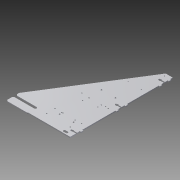
# Autodesk Inventor part: side_frame_v2
Saved by Autodesk Inventor 2013 (Build 170138000, 138)
## iProperties
Created: 2013-11-17
Part Number: side_frame_v2
Material: Generic
Document SubType Name: Modeling
Designer: Masta
Density: 1 g/cm^3
Author: Masta
Autodesk Inventor part; units mm, degrees
ref_plane "YZ Plane" through (0, 0, 0) normal (1, 0, 0) x (0, 1, 0)
ref_plane "XZ Plane" through (0, 0, 0) normal (0, 1, 0) x (-1, 0, 0)
ref_plane "XY Plane" through (0, 0, 0) normal (0, 0, 1) x (1, 0, 0)
sketch "Sketch1" plane through (0, 0, 0) normal (0, 0, 1) x (1, 0, 0)
  line L0 (255.7808, 350.0828) -> (255.7808, 358.8828)
  line L1 (251.6808, 67.29) -> (255.7808, 67.29)
  line L2 (255.7808, 67.29) -> (255.7808, 76.09)
  line L3 (255.7808, 76.09) -> (251.6808, 76.09)
  line L4 (251.6808, 76.09) -> (251.6808, 194.9901)
  line L5 (251.6808, 32.5401) -> (100.8808, 32.5401)
  line L6 (231.7439, 44.5401) -> (223.7479, 44.5401)
  line L7 (230.5808, 213.3401) -> (234.5808, 213.3401)
  line L8 (234.5808, 211.5401) -> (239.6808, 211.5401)
  line L9 (251.6808, 57.7345) -> (239.6808, 57.7345)
  line L10 (239.6808, 57.7345) -> (239.6808, 59.5345)
  line L11 (230.5808, 53.3345) -> (234.5808, 53.3345)
  line L12 (234.5808, 51.5345) -> (239.6808, 51.5345)
  line L13 (239.6808, 59.5345) -> (234.5808, 59.5345)
  line L14 (234.5808, 53.3345) -> (234.5808, 51.5345)
  line L15 (239.6808, 53.3345) -> (251.6808, 53.3345)
  line L16 (239.6808, 51.5345) -> (239.6808, 53.3345)
  line L17 (251.6808, 57.7345) -> (251.6808, 67.29)
  line L18 (251.6808, 217.7401) -> (239.6808, 217.7401)
  line L19 (255.7808, 236.0901) -> (251.6808, 236.0901)
  line L20 (251.6808, 236.0901) -> (251.6808, 350.0828)
  line L21 (255.7808, 203.7901) -> (251.6808, 203.7901)
  line L22 (251.6808, 194.9901) -> (255.7808, 194.9901)
  line L23 (255.7808, 194.9901) -> (255.7808, 203.7901)
  line L24 (251.6808, 227.2901) -> (251.6808, 217.7401)
  line L25 (251.6808, 213.3401) -> (251.6808, 203.7901)
  line L26 (251.6808, 382.3828) -> (255.7808, 382.3828)
  line L27 (255.7808, 382.3828) -> (255.7808, 391.1828)
  line L28 (255.7808, 391.1828) -> (251.6808, 391.1828)
  line L29 (251.6808, 391.1828) -> (251.6808, 400.5401)
  line L30 (255.7808, 358.8828) -> (251.6808, 358.8828)
  line L31 (251.6808, 350.0828) -> (255.7808, 350.0828)
  line L32 (73.8808, 35.5401) -> (73.8808, 51.1401)
  line L33 (239.6808, 211.5401) -> (239.6808, 213.3401)
  line L34 (230.5808, 217.7401) -> (230.5808, 213.3401)
  line L35 (73.8808, 77.5401) -> (226.2808, 400.5401)
  line L36 (234.5808, 217.7401) -> (230.5808, 217.7401)
  line L37 (234.5808, 217.7401) -> (234.5808, 219.5401)
  line L38 (251.6808, 400.5401) -> (226.2808, 400.5401)
  line L39 (239.6808, 213.3401) -> (251.6808, 213.3401)
  line L40 (231.7439, 36.5395) -> (223.7482, 36.5395)
  line L41 (239.6808, 219.5401) -> (234.5808, 219.5401)
  line L42 (98.8808, 30.5401) -> (78.8808, 30.5401)
  line L43 (234.5808, 213.3401) -> (234.5808, 211.5401)
  line L44 (230.5808, 372.825) -> (230.5808, 368.425)
  line L45 (234.5808, 372.825) -> (230.5808, 372.825)
  line L46 (234.5808, 372.825) -> (234.5808, 374.625)
  line L47 (251.6808, 372.825) -> (239.6808, 372.825)
  line L48 (230.5808, 368.425) -> (234.5808, 368.425)
  line L49 (239.6808, 368.425) -> (251.6808, 368.425)
  line L50 (234.5808, 366.625) -> (239.6808, 366.625)
  line L51 (239.6808, 374.625) -> (234.5808, 374.625)
  line L52 (234.5808, 368.425) -> (234.5808, 366.625)
  line L53 (251.6808, 372.825) -> (251.6808, 382.3828)
  line L54 (251.6808, 368.425) -> (251.6808, 358.8828)
  line L55 (230.5808, 57.7345) -> (230.5808, 53.3345)
  line L56 (234.5808, 57.7345) -> (230.5808, 57.7345)
  line L57 (234.5808, 57.7345) -> (234.5808, 59.5345)
  line L58 (239.6808, 366.625) -> (239.6808, 368.425)
  line L59 (239.6808, 372.825) -> (239.6808, 374.625)
  line L60 (78.8808, 56.1401) -> (148.8808, 56.1401)
  line L61 (78.8808, 56.1401) -> (73.8808, 51.1401)
  line L62 (78.8808, 64.9401) -> (148.8808, 64.9401)
  line L63 (73.8808, 69.9401) -> (73.8808, 77.5401)
  line L64 (78.8808, 64.9401) -> (73.8808, 69.9401)
  line L65 (251.6808, 227.2901) -> (255.7808, 227.2901)
  line L66 (255.7808, 227.2901) -> (255.7808, 236.0901)
  line L67 (239.6808, 217.7401) -> (239.6808, 219.5401)
  line L68 (78.8808, 30.5401) -> (73.8808, 35.5401)
  line L69 (100.8808, 32.5401) -> (98.8808, 30.5401)
  line L70 (251.6808, 32.5401) -> (251.6808, 53.3345)
  line L71 (136.6808, 189.5401) -> (231.6808, 189.5401) construction
  line L72 (231.6808, 189.5401) -> (231.6808, 93.5401) construction
  line L73 (231.6808, 93.5401) -> (136.6808, 93.5401) construction
  line L74 (136.6808, 93.5401) -> (136.6808, 189.5401) construction
  line L75 (164.6808, 93.5401) -> (208.6808, 93.5401) construction
  line L76 (208.6808, 93.5401) -> (208.6808, 187.5401) construction
  line L77 (208.6808, 187.5401) -> (164.6808, 187.5401) construction
  line L78 (164.6808, 187.5401) -> (164.6808, 93.5401) construction
  line L79 (160.3808, 93.5401) -> (208.6808, 93.5401) construction
  line L80 (208.6808, 93.5401) -> (208.6808, 168.5401) construction
  line L81 (208.6808, 168.5401) -> (160.3808, 168.5401) construction
  line L82 (160.3808, 168.5401) -> (160.3808, 93.5401) construction
  line L83 (208.6808, 168.5401) -> (208.6808, 174.8401) construction
  arc A0 (148.8808, 56.1401) -> (148.8808, 64.9401) centre (148.8808, 60.5401) ccw
  arc A1 (231.7439, 36.5395) -> (231.7439, 44.5401) centre (231.7439, 40.5398) ccw
  arc A2 (223.7479, 44.5401) -> (223.7482, 36.5395) centre (223.7482, 40.5398) ccw
  point P0 (0, 0)
  point P1 (219.7479, 40.5401)
  dimension "d0" = 177.8
  dimension "d9" = 95
  dimension "d10" = 96
  dimension "d11" = 44
  dimension "d12" = 94
  dimension "d15" = 48.3
  dimension "d16" = 75
  dimension "d18" = 6.3
  dimension "d19" = 23
  dimension "d20" = 20
  dimension "d21" = 63
  dimension "d22" = 4.1
  dimension "d23" = 8.8
  constraints: 168 end point, 17 collinear, 11 coincident, 7 parallel, 7 point on circle, 5 tangent, 4 horizontal, 3 centre point, 3 perpendicular, 1 vertical
  measures "d0" distance between parallel lines of L32 L70
  measures "d9" distance of L72.end L73.end
  measures "d10" distance of L71.end L72.end
  measures "d11" distance of L77.end L76.end
  measures "d12" distance of L75.end L76.end
  measures "d15" distance of L81.end L80.end
  measures "d16" distance of L80.end L75.end
  measures "d18" distance of L80.end L83.end
  measures "d19" distance between parallel lines of L72 L80
  measures "d20" distance between parallel lines of L4 L72
  measures "d21" distance between parallel lines of L42 L73
  measures "d22" distance between parallel lines of L2 L17
  measures "d23" distance of L1.end L2.end
extrude "Extrusion1" add sketch "Sketch1" against normal blind 4
hole "Hole1" at (136.6808, 189.5401, 0) at (136.6808, 93.5401, 0) at (231.6808, 93.5401, 0) at (231.6808, 189.5401, 0) at (160.3808, 93.5401, 0) at (208.6808, 93.5401, 0) at (208.6808, 174.8401, 0) at (160.3808, 168.5401, 0) at (164.6808, 93.5401, 0) at (164.6808, 187.5401, 0) at (208.6808, 187.5401, 0) direction (0, 0, -1) diameter 3.6 end through all
sketch "Sketch2" plane through (0, 0, 0) normal (0, 0, 1) x (1, 0, 0)
  line L0 (78.8808, 64.9401) -> (148.8808, 64.9401) projected
  line L1 (251.6808, 76.09) -> (251.6808, 194.9901) projected
  line L2 (162.1808, 84.5401) -> (212.1808, 84.5401) construction
  line L3 (212.1808, 84.5401) -> (212.1808, 234.5401) construction
  line L4 (212.1808, 234.5401) -> (162.1808, 234.5401) construction
  line L5 (162.1808, 234.5401) -> (162.1808, 84.5401) construction
  line L6 (162.1808, 84.5401) -> (212.1808, 234.5401) construction
  line L7 (212.1808, 84.5401) -> (162.1808, 234.5401) construction
  line L8 (129.6808, 49.5401) -> (244.6808, 49.5401) construction
  line L9 (244.6808, 49.5401) -> (244.6808, 269.5401) construction
  line L10 (244.6808, 269.5401) -> (129.6808, 269.5401) construction
  line L11 (129.6808, 269.5401) -> (129.6808, 49.5401) construction
  line L12 (129.6808, 49.5401) -> (244.6808, 269.5401) construction
  line L13 (244.6808, 49.5401) -> (129.6808, 269.5401) construction
  line L14 (223.7479, 44.5401) -> (231.7439, 44.5401) projected
  point P0 (0, 0)
  point P1 (187.1808, 159.5401)
  point P2 (187.1808, 159.5401)
  dimension "d33" = 50
  dimension "d34" = 150
  dimension "d35" = 115
  dimension "d36" = 220
  dimension "d38" = 7
  dimension "d82" = 5
  constraints: 24 end point, 5 midpoint, 4 coincident, 4 parallel, 2 horizontal, 2 perpendicular
  measures "d33" distance of L4.end L3.end
  measures "d34" distance of L3.end L2.end
  measures "d35" distance of L10.end L9.end
  measures "d36" distance of L9.end L8.end
  measures "d38" distance between parallel lines of L1 L9
  measures "d82" distance between parallel lines of L14 L8
hole "Hole2" at (162.1808, 234.5401, 0) at (162.1808, 84.5401, 0) at (212.1808, 84.5401, 0) at (212.1808, 234.5401, 0) direction (0, 0, -1) diameter 4.6 end through all
sketch "Sketch3" plane through (0, 0, 0) normal (0, 0, 1) x (1, 0, 0)
  line L0 (226.2808, 400.5401) -> (73.8808, 77.5401) projected
  line L1 (73.8808, 77.5401) -> (73.8808, 69.9401) projected
  line L2 (73.8808, 69.9401) -> (78.8808, 64.9401) projected
  line L3 (78.8808, 56.1401) -> (73.8808, 51.1401) projected
  line L4 (73.8808, 51.1401) -> (73.8808, 35.5401) projected
  line L5 (73.8808, 35.5401) -> (78.8808, 30.5401) projected
  line L6 (98.8808, 30.5401) -> (100.8808, 32.5401) projected
  line L7 (78.8808, 64.9401) -> (28.8808, 64.9401)
  line L8 (28.8808, 64.9401) -> (23.8808, 69.9401)
  line L9 (23.8808, 77.5401) -> (23.8808, 69.9401)
  line L10 (23.8808, 77.5401) -> (226.2808, 400.5401)
  line L11 (78.8808, 56.1401) -> (28.8808, 56.1401)
  line L12 (28.8808, 56.1401) -> (23.8808, 51.1401)
  line L13 (23.8808, 51.1401) -> (23.8808, 35.5401)
  line L14 (78.8808, 30.5401) -> (28.8808, 30.5401)
  line L15 (23.8808, 35.5401) -> (28.8808, 30.5401)
  point P0 (0, 0)
  point P1 (251.6808, 67.29)
  point P2 (251.6808, 76.09)
  point P3 (251.6808, 194.9901)
  point P4 (251.6808, 203.7901)
  point P5 (251.6808, 227.2901)
  point P6 (251.6808, 236.0901)
  point P7 (251.6808, 350.0828)
  point P8 (251.6808, 358.8828)
  point P9 (251.6808, 382.3828)
  point P10 (251.6808, 391.1828)
  dimension "d46" = 50
  dimension "d47" = 5
  dimension "d48" = 7.6
  constraints: 18 end point, 7 perpendicular
  measures "d46" distance of L2.end L7.end
  measures "d47" horizontal distance of L7.end L8.end
  measures "d48" distance of L9.start L8.end
extrude "Extrusion2" add sketch "Sketch3" against normal up to surface (4 mm away)
hole "Hole3" at (251.6808, 67.29, 0) at (251.6808, 76.09, 0) at (251.6808, 194.9901, 0) at (251.6808, 203.7901, 0) at (251.6808, 227.2901, 0) at (251.6808, 236.0901, 0) at (251.6808, 350.0828, 0) at (251.6808, 358.8828, 0) at (251.6808, 382.3828, 0) at (251.6808, 391.1828, 0) direction (0, 0, -1) diameter 1 end through all
sketch "Sketch5" plane through (0, 0, 0) normal (0, 0, 1) x (1, 0, 0)
  line L0 (251.6808, 53.3345) -> (239.6808, 53.3345) projected
  line L1 (239.6808, 53.3345) -> (239.6808, 51.5345) projected
  line L2 (239.6808, 51.5345) -> (234.5808, 51.5345) projected
  line L3 (234.5808, 51.5345) -> (234.5808, 53.3345) projected
  line L4 (234.5808, 53.3345) -> (230.5808, 53.3345) projected
  line L5 (230.5808, 53.3345) -> (230.5808, 57.7345) projected
  line L6 (230.5808, 57.7345) -> (234.5808, 57.7345) projected
  line L7 (234.5808, 57.7345) -> (234.5808, 59.5345) projected
  line L8 (234.5808, 59.5345) -> (239.6808, 59.5345) projected
  line L9 (239.6808, 59.5345) -> (239.6808, 57.7345) projected
  line L10 (239.6808, 57.7345) -> (251.6808, 57.7345) projected
  line L11 (251.6808, 213.3401) -> (239.6808, 213.3401) projected
  line L12 (239.6808, 213.3401) -> (239.6808, 211.5401) projected
  line L13 (239.6808, 211.5401) -> (234.5808, 211.5401) projected
  line L14 (234.5808, 211.5401) -> (234.5808, 213.3401) projected
  line L15 (234.5808, 213.3401) -> (230.5808, 213.3401) projected
  line L16 (230.5808, 213.3401) -> (230.5808, 217.7401) projected
  line L17 (230.5808, 217.7401) -> (234.5808, 217.7401) projected
  line L18 (234.5808, 217.7401) -> (234.5808, 219.5401) projected
  line L19 (234.5808, 219.5401) -> (239.6808, 219.5401) projected
  line L20 (239.6808, 219.5401) -> (239.6808, 217.7401) projected
  line L21 (239.6808, 217.7401) -> (251.6808, 217.7401) projected
  line L22 (251.6808, 368.425) -> (239.6808, 368.425) projected
  line L23 (239.6808, 368.425) -> (239.6808, 366.625) projected
  line L24 (239.6808, 366.625) -> (234.5808, 366.625) projected
  line L25 (234.5808, 366.625) -> (234.5808, 368.425) projected
  line L26 (234.5808, 368.425) -> (230.5808, 368.425) projected
  line L27 (230.5808, 368.425) -> (230.5808, 372.825) projected
  line L28 (230.5808, 372.825) -> (234.5808, 372.825) projected
  line L29 (234.5808, 372.825) -> (234.5808, 374.625) projected
  line L30 (234.5808, 374.625) -> (239.6808, 374.625) projected
  line L31 (239.6808, 374.625) -> (239.6808, 372.825) projected
  line L32 (239.6808, 372.825) -> (251.6808, 372.825) projected
  line L33 (231.7439, 36.5395) -> (223.7482, 36.5395) projected
  line L34 (251.6808, 217.7401) -> (251.6808, 213.3401)
  line L35 (251.6808, 368.425) -> (251.6808, 372.825)
  line L36 (251.6808, 53.3345) -> (251.6808, 57.7345)
  line L37 (28.8808, 64.9401) -> (148.8808, 64.9401) projected
  arc A0 (148.8808, 56.1401) -> (148.8808, 64.9401) centre (148.8808, 60.5401) ccw projected
  line L38 (148.8808, 56.1401) -> (28.8808, 56.1401) projected
  arc A1 (98.8808, 56.1401) -> (98.8808, 64.9401) centre (98.8808, 60.5401) ccw
  point P0 (0, 0)
  point P1 (251.6808, 215.5401)
  point P2 (251.6808, 370.625)
  point P3 (251.6808, 55.5345)
  dimension "d85" = 50
  constraints: 6 end point, 3 midpoint, 2 collinear, 2 point on circle, 2 point on line, 2 tangent, 1 centre point, 1 perpendicular
  measures "d85" distance of A0.centre A1.centre
extrude "Extrusion3" add sketch "Sketch5" against normal up to surface (4 mm away)
sketch "Sketch6" plane through (0, 0, 0) normal (0, 0, 1) x (1, 0, 0)
  line L0 (251.6808, 204.2901) -> (251.6808, 226.7901) projected
  line L1 (231.7439, 36.5395) -> (223.7482, 36.5395) projected
  line L2 (251.6808, 215.5401) -> (230.6808, 215.5401) construction
  line L3 (239.6808, 213.5401) -> (251.6808, 213.5401)
  line L4 (251.6808, 213.5401) -> (251.6808, 217.5401)
  line L5 (251.6808, 217.5401) -> (239.6808, 217.5401)
  line L6 (239.6808, 217.5401) -> (239.6808, 213.5401)
  line L7 (239.6808, 213.5401) -> (251.6808, 217.5401) construction
  line L8 (251.6808, 213.5401) -> (239.6808, 217.5401) construction
  line L9 (234.6808, 212.0901) -> (239.6808, 212.0901)
  line L10 (239.6808, 212.0901) -> (239.6808, 218.9901)
  line L11 (239.6808, 218.9901) -> (234.6808, 218.9901)
  line L12 (234.6808, 218.9901) -> (234.6808, 212.0901)
  line L13 (234.6808, 212.0901) -> (239.6808, 218.9901) construction
  line L14 (239.6808, 212.0901) -> (234.6808, 218.9901) construction
  line L15 (230.6808, 213.5401) -> (234.6808, 213.5401)
  line L16 (234.6808, 213.5401) -> (234.6808, 217.5401)
  line L17 (234.6808, 217.5401) -> (230.6808, 217.5401)
  line L18 (230.6808, 217.5401) -> (230.6808, 213.5401)
  line L19 (230.6808, 213.5401) -> (234.6808, 217.5401) construction
  line L20 (234.6808, 213.5401) -> (230.6808, 217.5401) construction
  point P0 (0, 0)
  point P1 (245.6808, 215.5401)
  point P2 (237.1808, 215.5401)
  point P3 (232.6808, 215.5401)
  dimension "d62" = 21
  dimension "d63" = 4
  dimension "d64" = 5
  dimension "d65" = 12
  dimension "d66" = 6.9
  constraints: 38 end point, 7 midpoint, 7 parallel, 6 coincident, 5 point on line, 3 horizontal, 3 perpendicular, 2 collinear
  measures "d62" distance of L2.start L2.end
  measures "d63" distance between parallel lines of L3 L5
  measures "d64" distance of L10.end L11.end
  measures "d65" distance of L4.end L5.end
  measures "d66" distance between parallel lines of L9 L11
extrude "Extrusion4" cut sketch "Sketch6" against normal up to surface (4 mm away)
hole "Hole4" at (251.6808, 215.5401, 0) at (234.6808, 218.9901, 0) at (230.6808, 217.5401, 0) at (230.6808, 213.5401, 0) at (239.6808, 218.9901, 0) at (234.6808, 212.0901, 0) at (239.6808, 212.0901, 0) direction (0, 0, -1) diameter 1 end through all
pattern_linear "Rectangular Pattern1" count 2 spacing 155 along (0, 1, 0) of "Hole4", "Extrusion4"
pattern_linear "Rectangular Pattern2" count 2 spacing 160 along (0, -1, 0) of "Hole4", "Extrusion4"
sketch "Sketch7" plane through (0, 0, 0) normal (0, 0, 1) x (1, 0, 0)
  circle A0 centre (136.6808, 189.5401) radius 1.8 projected
  line L0 (129.6808, 269.5401) -> (129.6808, 49.5401) construction
  line L1 (244.6808, 269.5401) -> (129.6808, 269.5401) construction
  line L2 (244.6808, 49.5401) -> (244.6808, 269.5401) construction
  line L3 (129.6808, 49.5401) -> (244.6808, 49.5401) construction
  line L4 (136.6808, 63.5401) -> (221.6808, 63.5401) construction
  line L5 (221.6808, 63.5401) -> (221.6808, 189.5401) construction
  line L6 (221.6808, 189.5401) -> (136.6808, 189.5401) construction
  line L7 (136.6808, 189.5401) -> (136.6808, 63.5401) construction
  line L8 (251.6808, 236.5901) -> (251.6808, 349.5828) projected
  line L9 (251.6808, 400.5401) -> (226.2808, 400.5401) projected
  line L10 (241.6808, 395.5401) -> (181.6808, 395.5401) construction
  line L11 (181.6808, 395.5401) -> (181.6808, 293.5401) construction
  line L12 (181.6808, 293.5401) -> (241.6808, 293.5401) construction
  line L13 (241.6808, 293.5401) -> (241.6808, 395.5401) construction
  line L14 (232.1808, 390.5401) -> (232.1808, 307.5401) construction
  point P0 (0, 0)
  point P1 (183.8808, 308.5401)
  dimension "d86" = 85
  dimension "d87" = 126
  dimension "d95" = 60
  dimension "d96" = 102
  dimension "d97" = 5
  dimension "d98" = 10
  dimension "d99" = 9.5
  dimension "d100" = 5
  dimension "d101" = 14
  dimension "d102" = 15
  dimension "d103" = 48.3
  constraints: 18 end point, 6 coincident, 5 parallel, 2 horizontal, 2 perpendicular
  measures "d86" distance of L4.start L4.end
  measures "d87" distance of L6.end L4.start
  measures "d95" distance of L10.start L10.end
  measures "d96" distance of L10.end L11.end
  measures "d97" distance between parallel lines of L10 L9
  measures "d98" distance between parallel lines of L13 L8
  measures "d99" distance between parallel lines of L13 L14
  measures "d100" distance from line of L10 L14.start
  measures "d101" distance from line of L12 L14.end
  measures "d102" distance from line of L12 point (183.881, 308.54)
  measures "d103" horizontal distance of point (232.181, 307.54) point (183.881, 308.54)
hole "Hole5" at (136.6808, 63.5401, 0) at (221.6808, 63.5401, 0) at (221.6808, 189.5401, 0) direction (0, 0, -1) diameter 3.6 end through all
hole "Hole6" at (183.8808, 308.5401, 0) at (232.1808, 307.5401, 0) at (232.1808, 390.5401, 0) direction (0, 0, -1) diameter 3 end through all
body "Solid1"
